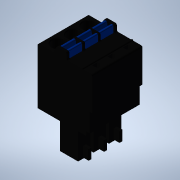
# Autodesk Inventor part: 8079508 3GD-1RR3.5-CLP-CBL---(2)
Saved by Autodesk Inventor 2021 (Build 250183000, 183)
## iProperties
Created: 2026-04-23
Part Number: 8079508 3GD-1RR3.5-CLP-CBL---(2)
Material: Generic
Catalog Web Link: www.3dfindit.com
Description: NEKM-C-5---(2)-assortment of plugs
Vendor: FESTO
Document SubType Name: Modeling
Designer: psAdmin
Manufacturer: FESTO
Mass: 1.89316 g
Surface Area: 14.2046 cm^2
Volume: 1.89316 cm^3
Density: 1 g/cm^3
Appearance: PSOLRGB-79-79-79
Category: PARTsolutions
Company: FESTO
Title: 8079508 3GD-1RR3.5-CLP-CBL---(2)
Author: Cadenas PARTsolutions
Comments: assortment of plugs
PSOL_IDENT_0: {$CADENAS_DATA/23d-libs/festo/parts/n/nekm/parts/nekm_p2.prj},213 {VTYP=3D},{NB=8079508 3GD-1RR3.5-C
PSOL_IDENT_1: LP-CBL---(2)},{LINA=8079508 3GD-1RR3.5-CLP-CBL---(2)},{NN=NEKM-C-5---(2)},{DATE=05.12.2025 12:36:19}
PSOL_IDENT_2: ,{GEOMDATE=30.08.2023 11:07:56},{VERSION=},{LINEID=250},{WBVAR=},{WBNUMERIC=}  {NB=8079508 3GD-1RR3.
PSOL_IDENT_3: 5-CLP-CBL---(2)},{LINA=8079508 3GD-1RR3.5-CLP-CBL---(2)},{KT=DUMMY},{TNR=8079508},{TYP=3GD-1RR3.5-CL
PSOL_IDENT_4: P-CBL},{V=10.000},{ZZ=3.000}
NB: 8079508 3GD-1RR3.5-CLP-CBL---(2)
NN: NEKM-C-5---(2)
NT: assortment of plugs
NBSYN: $TNR. $TYP.---(2)
LINA: 8079508 3GD-1RR3.5-CLP-CBL---(2)
CATALOG: Festo
TNR: 8079508
TYP: 3GD-1RR3.5-CLP-CBL
V: 10
ZZ: 3
SUPPLIER: FESTO
ARTICLENO: 8079508 3GD-1RR3.5-CLP-CBL---(2)
BOMINFO: 8079508 3GD-1RR3.5-CLP-CBL---(2)
CREATOR: CADENAS GmbH
Autodesk Inventor part; units mm, degrees
sketch "Sketch_1" plane through (0, 0, 0) normal (0, 0, 1) x (1, 0, 0)
  line L0 (0, 12.4) -> (0, 0)
  line L1 (0, 0) -> (10.8, 0)
  arc A0 (10.8, 0) -> (11.1, 0.3) centre (10.8, 0.3) ccw
  line L2 (11.1, 0.3) -> (11.1, 0.9)
  line L3 (11.1, 0.9) -> (11.8, 0.9)
  line L4 (11.8, 0.9) -> (11.8, 5.112)
  line L5 (11.8, 5.112) -> (12.4, 5.112)
  line L6 (12.4, 5.112) -> (12.4, 12.4)
  arc A1 (12.4, 12.4) -> (12.1, 12.7) centre (12.1, 12.4) ccw
  line L7 (12.1, 12.7) -> (10.3, 12.7)
  arc A2 (10.3, 12.7) -> (9.9, 12.7) centre (10.1, 12.7) ccw
  line L8 (9.9, 12.7) -> (6.9, 12.7)
  arc A3 (6.6, 13) -> (6.9, 12.7) centre (6.9, 13) ccw
  line L9 (6.6, 13) -> (6.6, 13.9)
  arc A4 (6.6, 13.9) -> (6.3, 14.2) centre (6.3, 13.9) ccw
  line L10 (6.3, 14.2) -> (4.4906, 14.2)
  arc A5 (4.4906, 14.2) -> (4.2187, 14.0268) centre (4.4906, 13.9) ccw
  line L11 (4.2187, 14.0268) -> (3.6808, 12.8732)
  arc A6 (3.4089, 12.7) -> (3.6808, 12.8732) centre (3.4089, 13) ccw
  line L12 (3.4089, 12.7) -> (0.3, 12.7)
  arc A7 (0.3, 12.7) -> (0, 12.4) centre (0.3, 12.4) ccw
  constraints: 26 end point, 16 point on circle, 8 centre point
extrude "Extrusion1" add sketch "Sketch_1" against normal blind 11.4
sketch "Sketch_4" plane through (0, 0, 0) normal (0, 1, 0) x (-1, 0, 0)
  line L0 (-8.5, -10.7) -> (-8.5, -0.7)
  line L1 (-8.5, -0.7) -> (-18.5, -0.7)
  line L2 (-18.5, -0.7) -> (-18.5, -10.7)
  line L3 (-18.5, -10.7) -> (-8.5, -10.7)
  constraints: 8 end point
extrude "Extrusion2" cut sketch "Sketch_4" along normal blind 0.9
sketch "Sketch_20" plane through (0, 0, 0) normal (0, 1, 0) x (-1, 0, 0)
  line L0 (-4.4, -1.1513) -> (-4.4, -0.7)
  line L1 (-4.4, -0.7) -> (-8.5, -0.7)
  line L2 (-8.5, -0.7) -> (-8.5, -3.5)
  line L3 (-8.5, -3.5) -> (-4.4, -3.5)
  line L4 (-4.4, -3.5) -> (-4.4, -3.0487)
  arc A0 (-4.4, -1.1513) -> (-4.4, -3.0487) centre (-3.05, -2.1) ccw
  constraints: 10 end point, 2 point on circle, 1 centre point
extrude "Extrusion3" add sketch "Sketch_20" against normal blind 6.6
pattern_linear "Rectangular Pattern1" count 3 spacing 3.5 along (0, 0, -1) of "Extrusion3"
sketch "Sketch_5" plane through (0, -6.35, 0) normal (0, 1, 0) x (1, 0, 0)
  line L0 (6.5, 2.5) -> (6.5, 1.8)
  line L1 (6.5, 1.8) -> (9.7, 1.8)
  arc A0 (9.7, 1.8) -> (9.8, 1.9) centre (9.7, 1.9) ccw
  line L2 (9.8, 1.9) -> (9.8, 2.4)
  arc A1 (9.8, 2.4) -> (9.7, 2.5) centre (9.7, 2.4) ccw
  line L3 (9.7, 2.5) -> (6.5, 2.5)
  constraints: 8 end point, 4 point on circle, 2 centre point
extrude "Extrusion4" add sketch "Sketch_5" along normal blind 2.25
pattern_linear "Rectangular Pattern2" count 3 spacing 3.5 along (0, 0, -1) of "Extrusion4"
sketch "Sketch_6" plane through (0, 0, 0) normal (1, 0, 0) x (0, 1, 0)
  line L0 (17.7, -0.6) -> (12.7, -0.6)
  line L1 (12.7, -0.6) -> (12.7, -3.7)
  line L2 (12.7, -3.7) -> (17.7, -3.7)
  line L3 (17.7, -3.7) -> (17.7, -0.6)
  constraints: 8 end point
extrude "Extrusion5" cut sketch "Sketch_6" along normal blind 8
sketch "Pattern_5_SKETCH_1" plane through (0, 0, -3.6) normal (1, 0, 0) x (0, 0, -1)
  line L0 (0.6, 17.7) -> (0.6, 12.7)
  line L1 (0.6, 12.7) -> (3.7, 12.7)
  line L2 (3.7, 12.7) -> (3.7, 17.7)
  line L3 (3.7, 17.7) -> (0.6, 17.7)
  constraints: 8 end point
sketch "Pattern_5_SKETCH_2" plane through (0, 0, -7.1) normal (1, 0, 0) x (0, 0, -1)
  line L0 (0.6, 17.7) -> (0.6, 12.7)
  line L1 (0.6, 12.7) -> (3.7, 12.7)
  line L2 (3.7, 12.7) -> (3.7, 17.7)
  line L3 (3.7, 17.7) -> (0.6, 17.7)
  constraints: 8 end point
extrude "Extrusion6" cut sketch "Pattern_5_SKETCH_1" along normal blind 8
extrude "Extrusion7" cut sketch "Pattern_5_SKETCH_2" along normal blind 8
sketch "Sketch_7" plane through (4.45, 0, 0) normal (1, 0, 0) x (0, 0, -1)
  line L0 (0.6, 17.6) -> (0.6, 12.6)
  line L1 (0.6, 12.6) -> (3.7, 12.6)
  line L2 (3.7, 12.6) -> (3.7, 17.6)
  line L3 (3.7, 17.6) -> (0.6, 17.6)
  constraints: 8 end point
extrude "Extrusion8" cut sketch "Sketch_7" along normal blind 2.15
sketch "Pattern_6_SKETCH_1" plane through (4.45, 0, 0) normal (1, 0, 0) x (0, 0, -1)
  line L0 (4.2, 17.6) -> (4.2, 12.6)
  line L1 (4.2, 12.6) -> (7.3, 12.6)
  line L2 (7.3, 12.6) -> (7.3, 17.6)
  line L3 (7.3, 17.6) -> (4.2, 17.6)
  constraints: 8 end point
sketch "Pattern_6_SKETCH_2" plane through (4.45, 0, 0) normal (1, 0, 0) x (0, 0, -1)
  line L0 (7.7, 17.6) -> (7.7, 12.6)
  line L1 (7.7, 12.6) -> (10.8, 12.6)
  line L2 (10.8, 12.6) -> (10.8, 17.6)
  line L3 (10.8, 17.6) -> (7.7, 17.6)
  constraints: 8 end point
extrude "Extrusion9" cut sketch "Pattern_6_SKETCH_1" along normal blind 2.15
extrude "Extrusion10" cut sketch "Pattern_6_SKETCH_2" along normal blind 2.15
sketch "Sketch_8" plane through (0, 0, -0.65) normal (0, 0, 1) x (1, 0, 0)
  line L0 (4.45, 14) -> (4.45, 12.6)
  line L1 (4.45, 12.6) -> (6.45, 12.6)
  line L2 (6.45, 12.6) -> (6.45, 14)
  arc A0 (6.45, 14) -> (6.25, 14.2) centre (6.25, 14) ccw
  line L3 (6.25, 14.2) -> (6.1353, 14.2)
  arc A1 (6.1353, 14.2) -> (5.8912, 14.0041) centre (6.1353, 13.95) ccw
  line L4 (5.8912, 14.0041) -> (5.7429, 13.3351)
  arc A2 (5.1571, 13.3351) -> (5.7429, 13.3351) centre (5.45, 13.4) ccw
  line L5 (5.1571, 13.3351) -> (5.0088, 14.0041)
  arc A3 (5.0088, 14.0041) -> (4.7647, 14.2) centre (4.7647, 13.95) ccw
  line L6 (4.7647, 14.2) -> (4.65, 14.2)
  arc A4 (4.65, 14.2) -> (4.45, 14) centre (4.65, 14) ccw
  constraints: 14 end point, 10 point on circle, 5 centre point
extrude "Extrusion11" add sketch "Sketch_8" against normal blind 3
sketch "Pattern_1_SKETCH_1" plane through (0, 0, -4.25) normal (0, 0, 1) x (1, 0, 0)
  line L0 (4.45, 14) -> (4.45, 12.6)
  line L1 (4.45, 12.6) -> (6.45, 12.6)
  line L2 (6.45, 12.6) -> (6.45, 14)
  arc A0 (6.45, 14) -> (6.25, 14.2) centre (6.25, 14) ccw
  line L3 (6.25, 14.2) -> (6.1353, 14.2)
  arc A1 (6.1353, 14.2) -> (5.8912, 14.0041) centre (6.1353, 13.95) ccw
  line L4 (5.8912, 14.0041) -> (5.7429, 13.3351)
  arc A2 (5.1571, 13.3351) -> (5.7429, 13.3351) centre (5.45, 13.4) ccw
  line L5 (5.1571, 13.3351) -> (5.0088, 14.0041)
  arc A3 (5.0088, 14.0041) -> (4.7647, 14.2) centre (4.7647, 13.95) ccw
  line L6 (4.7647, 14.2) -> (4.65, 14.2)
  arc A4 (4.65, 14.2) -> (4.45, 14) centre (4.65, 14) ccw
  constraints: 14 end point, 10 point on circle, 5 centre point
sketch "Pattern_1_SKETCH_2" plane through (0, 0, -7.75) normal (0, 0, 1) x (1, 0, 0)
  line L0 (4.45, 14) -> (4.45, 12.6)
  line L1 (4.45, 12.6) -> (6.45, 12.6)
  line L2 (6.45, 12.6) -> (6.45, 14)
  arc A0 (6.45, 14) -> (6.25, 14.2) centre (6.25, 14) ccw
  line L3 (6.25, 14.2) -> (6.1353, 14.2)
  arc A1 (6.1353, 14.2) -> (5.8912, 14.0041) centre (6.1353, 13.95) ccw
  line L4 (5.8912, 14.0041) -> (5.7429, 13.3351)
  arc A2 (5.1571, 13.3351) -> (5.7429, 13.3351) centre (5.45, 13.4) ccw
  line L5 (5.1571, 13.3351) -> (5.0088, 14.0041)
  arc A3 (5.0088, 14.0041) -> (4.7647, 14.2) centre (4.7647, 13.95) ccw
  line L6 (4.7647, 14.2) -> (4.65, 14.2)
  arc A4 (4.65, 14.2) -> (4.45, 14) centre (4.65, 14) ccw
  constraints: 14 end point, 10 point on circle, 5 centre point
extrude "Extrusion12" add sketch "Pattern_1_SKETCH_1" against normal blind 3
extrude "Extrusion13" add sketch "Pattern_1_SKETCH_2" against normal blind 3
sketch "Sketch_10" plane through (2.4, 0, 0) normal (1, 0, 0) x (0, 0, -1)
  line L0 (2.45, 8.7) -> (2.45, 12.7)
  line L1 (2.45, 12.7) -> (4.1, 12.7)
  line L2 (4.1, 12.7) -> (4, 12.5268)
  line L3 (4, 12.5268) -> (4, 10.5)
  line L4 (4, 10.5) -> (3.2, 8.7844)
  line L5 (3.2, 8.7844) -> (3.2, 8.7)
  line L6 (3.2, 8.7) -> (2.45, 8.7)
  line L7 (2.45, 8.7) -> (2.45, 12.7)
  constraints: 16 end point
revolve "Revolution1" cut sketch "Sketch_10" angle 360 about axis through (2.4, 8.7, -2.45) along (0, -1, 0)
pattern_linear "Rectangular Pattern3" count 3 spacing 3.5 along (0, 0, -1) of "Revolution1"
sketch "Sketch_12" plane through (0, 12.7, 0) normal (0, 1, 0) x (1, 0, 0)
  line L0 (0.4, 4.4) -> (0.4, 4)
  line L1 (0.4, 4) -> (3.8, 4)
  line L2 (3.8, 4) -> (3.8, 4.4)
  line L3 (3.8, 4.4) -> (0.4, 4.4)
  constraints: 8 end point
extrude "Extrusion14" add sketch "Sketch_12" against normal blind 3.85
pattern_linear "Rectangular Pattern4" count 2 spacing 3.5 along (0, 0, -1) of "Extrusion14"
sketch "Sketch_13" plane through (0, 12.7, 0) normal (0, 1, 0) x (1, 0, 0)
  line L0 (10.5, 3) -> (10.5, 1.9)
  line L1 (10.5, 1.9) -> (11.05, 1.9)
  arc A0 (11.05, 1.9) -> (11.05, 3) centre (11.05, 2.45) ccw
  line L2 (11.05, 3) -> (10.5, 3)
  constraints: 6 end point, 2 point on circle, 1 centre point
extrude "Extrusion15" cut sketch "Sketch_13" against normal blind 3.7
pattern_linear "Rectangular Pattern5" count 3 spacing 3.5 along (0, 0, -1) of "Extrusion15"
sketch "Sketch_15" plane through (0, -5.6, 0) normal (0, 1, 0) x (1, 0, 0)
  circle A0 centre (6.6, 2.2) radius 0.8
  constraints: 1 centre point
extrude "Extrusion16" cut sketch "Sketch_15" against normal blind 2
pattern_linear "Rectangular Pattern6" count 2 spacing 3.5 along (0, 0, -1) of "Extrusion16"
sketch "Sketch_17" plane through (0, -5.6, 0) normal (0, 1, 0) x (1, 0, 0)
  arc A0 (5.9386, 9.65) -> (7.2614, 9.65) centre (6.6, 9.2) ccw
  line L0 (7.2614, 9.65) -> (5.9386, 9.65)
  constraints: 2 end point, 2 point on circle, 1 centre point
extrude "Extrusion17" cut sketch "Sketch_17" against normal blind 2
ref_plane "ANBAU_XY" through (6.2, 0, -5.7) normal (1, 0, 0) x (0, 0, -1)
ref_plane "ANBAU_YZ" through (6.2, 0, -5.7) normal (0, 0, -1) x (0, 1, 0)
ref_plane "ANBAU_ZX" through (6.2, 0, -5.7) normal (0, 1, 0) x (1, 0, 0)
ref_plane "CP1_XY" through (6.6, 0, -5.7) normal (0, 1, 0) x (1, 0, 0)
ref_plane "CP1_YZ" through (6.6, 0, -5.7) normal (1, 0, 0) x (0, 0, -1)
ref_plane "CP1_ZX" through (6.6, 0, -5.7) normal (0, 0, -1) x (0, 1, 0)
ref_plane "ECP_1_XY" through (2.4, 2.7, -9.45) normal (0, 1, 0) x (1, 0, 0)
ref_plane "ECP_1_YZ" through (2.4, 2.7, -9.45) normal (1, 0, 0) x (0, 0, -1)
ref_plane "ECP_1_ZX" through (2.4, 2.7, -9.45) normal (0, 0, -1) x (0, 1, 0)
ref_plane "ECP_2_XY" through (2.4, 2.7, -5.95) normal (0, 1, 0) x (1, 0, 0)
ref_plane "ECP_2_YZ" through (2.4, 2.7, -5.95) normal (1, 0, 0) x (0, 0, -1)
ref_plane "ECP_2_ZX" through (2.4, 2.7, -5.95) normal (0, 0, -1) x (0, 1, 0)
ref_plane "ECP_3_XY" through (2.4, 2.7, -2.45) normal (0, 1, 0) x (1, 0, 0)
ref_plane "ECP_3_YZ" through (2.4, 2.7, -2.45) normal (1, 0, 0) x (0, 0, -1)
ref_plane "ECP_3_ZX" through (2.4, 2.7, -2.45) normal (0, 0, -1) x (0, 1, 0)
ref_plane "IP1_XY" through (24, -6.6, -2.2) normal (0, 1, 0) x (1, 0, 0)
ref_plane "IP1_YZ" through (24, -6.6, -2.2) normal (1, 0, 0) x (0, 0, -1)
ref_plane "IP1_ZX" through (24, -6.6, -2.2) normal (0, 0, -1) x (0, 1, 0)
ref_plane "IP2_XY" through (4, -6.6, -17.95) normal (0, -1, 0) x (1, 0, 0)
ref_plane "IP2_YZ" through (4, -6.6, -17.95) normal (1, 0, 0) x (0, 0, 1)
ref_plane "IP2_ZX" through (4, -6.6, -17.95) normal (0, 0, 1) x (0, -1, 0)
ref_plane "MD_XY" through (6.6, -6.6, -9.2) normal (0, -1, 0) x (1, 0, 0)
ref_plane "MD_YZ" through (6.6, -6.6, -9.2) normal (1, 0, 0) x (0, 0, 1)
ref_plane "MD_ZX" through (6.6, -6.6, -9.2) normal (0, 0, 1) x (0, -1, 0)
ref_plane "NEKM_10_XY" through (6.6, -6.6, -2.2) normal (0, -1, 0) x (1, 0, 0)
ref_plane "NEKM_10_YZ" through (6.6, -6.6, -2.2) normal (1, 0, 0) x (0, 0, 1)
ref_plane "NEKM_10_ZX" through (6.6, -6.6, -2.2) normal (0, 0, 1) x (0, -1, 0)
ref_plane "OP_XY" through (12.4, -6.6, 0) normal (0, 1, 0) x (0, 0, -1)
ref_plane "OP_YZ" through (12.4, -6.6, 0) normal (0, 0, -1) x (-1, 0, 0)
ref_plane "OP_ZX" through (12.4, -6.6, 0) normal (-1, 0, 0) x (0, 1, 0)
body "Solid1"
